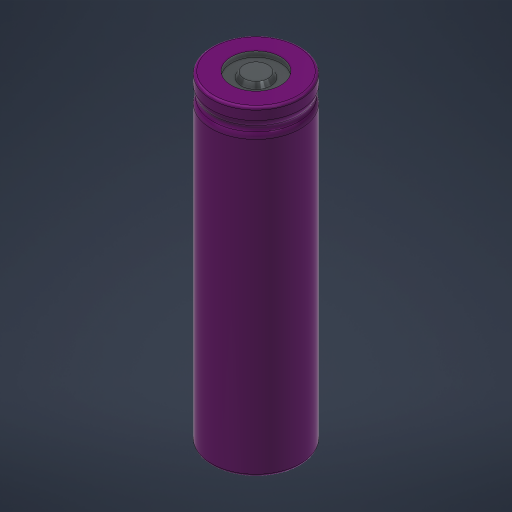
# Autodesk Inventor part: 18650
Saved by Autodesk Inventor 2024.3 (Build 283343010, 343A)
## iProperties
Created: 2025-03-19
Part Number: 18650
Material: Generisch
Document SubType Name: Modeling
Designer: David Lill
Density: 1 g/cm^3
Appearance: Zink
Author: David Lill
Autodesk Inventor part; units mm, degrees
ref_plane "YZ Plane" through (0, 0, 0) normal (1, 0, 0) x (0, 1, 0)
ref_plane "XZ Plane" through (0, 0, 0) normal (0, 1, 0) x (-1, 0, 0)
ref_plane "XY Plane" through (0, 0, 0) normal (0, 0, 1) x (1, 0, 0)
sketch "Skizze1" plane through (0, 0, 0) normal (0, 1, 0) x (-1, 0, 0)
  line L0 (0, 0) -> (7, 0)
  line L1 (7, 0) -> (7, -0.1)
  line L2 (7, -0.1) -> (8.5, -0.1)
  arc A0 (8.5, -0.1) -> (9, 0.4) centre (8.5, 0.4) ccw
  line L3 (9, 0.4) -> (9, 60.034)
  arc A1 (9, 61.766) -> (9, 60.034) centre (9.5, 60.9) ccw
  line L4 (9, 61.766) -> (9, 64.4)
  arc A2 (9, 64.4) -> (8.5, 64.9) centre (8.5, 64.4) ccw
  line L5 (8.5, 64.9) -> (5, 64.9)
  line L6 (5, 64.9) -> (5, 63.8)
  line L7 (5, 63.8) -> (3, 63.8)
  line L8 (3, 63.8) -> (2.4226, 64.8)
  line L9 (2.4226, 64.8) -> (0, 64.8)
  line L10 (0, 64.8) -> (0, 0)
  dimension "d4" = 18
  dimension "d5" = 1
  dimension "d6" = 19
  dimension "d7" = 0.5
  dimension "d8" = 0.1
  dimension "d9" = 14
  dimension "d10" = 1
  dimension "d11" = 10
  dimension "d12" = 6
  dimension "d13" = 4
  dimension "d14" = 60
  dimension "d17" = 0.1
  dimension "d18" = 65
  constraints: 22 end point, 7 perpendicular, 6 point on circle, 4 tangent, 3 centre point, 2 point on line, 1 equal radius, 1 horizontal
  measures "d4" diameter of L3 L10
  measures "d5" radius of A1
  measures "d6" diameter of A1.centre L10
  measures "d7" radius of A2
  measures "d8" distance between parallel lines of L0 L2
  measures "d9" diameter of L1 L10
  measures "d10" distance between parallel lines of L7 L9
  measures "d11" diameter of L6 L10
  measures "d12" diameter of L7.end L10
  measures "d13" distance from line of A1.centre L5
  measures "d14" angle of L7 L8
  measures "d17" distance between parallel lines of L9 L5
  measures "d18" distance between parallel lines of L2 L5
revolve "Umdrehung1" add sketch "Skizze1" angle 360 about axis through (0, 0, 64.8) along (0, 0, -1)
fillet "Rundung1" radius 2 2 edges at (9, 0, 60.034) (9, 0, 61.766)
equation "\"d17\" = d8"
